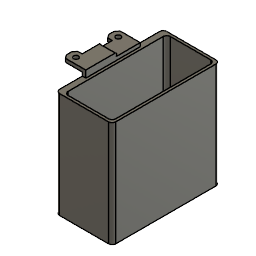
Mounting Bracke_bx_V2 (Autodesk Fusion 360 design; units mm, degrees)
Autodesk Fusion 360 part; units mm, degrees
sketch "Sketch1" plane through (0, 0, 0) normal (0, 1, 0) x (1, 0, 0)
  line L0 (0, 0) -> (0, 24)
  circle A0 centre (0, 24) radius 1.4
  circle A1 centre (0, 0) radius 1.4
  line L1 (0, 0) -> (0, -3.5)
  line L2 (0, 0) -> (0, 3.5)
  line L3 (0, -3.5) -> (-2.5, -3.5)
  line L4 (0, 3.5) -> (-2.5, 3.5)
  line L5 (-4, 0) -> (-4, 1.5)
  line L6 (-4, 0) -> (-4, -1.5)
  line L7 (-2.5, 3.5) -> (-4, 1.5)
  line L8 (-4, -1.5) -> (-2.5, -3.5)
  line L9 (0, 3.5) -> (0, 24)
  line L10 (0, 24) -> (0, 20.5)
  line L11 (0, 24) -> (5, 24)
  line L12 (5, 24) -> (5, 0)
  line L13 (5, 0) -> (0, 0)
  line L14 (5, 12) -> (0, 12)
  line L15 (-2.5, 20.5) -> (-4, 22.5)
  line L16 (0, 20.5) -> (-2.5, 20.5)
  line L17 (-4, 24) -> (-4, 22.5)
  line L18 (-4, 24) -> (-4, 25.5)
  line L19 (0, 27.5) -> (-2.5, 27.5)
  line L20 (-4, 25.5) -> (-2.5, 27.5)
  line L21 (0, -3.5) -> (5, -3.5)
  line L22 (5, -3.5) -> (5, 0)
  line L23 (0, 27.5) -> (5, 27.5)
  line L24 (5, 27.5) -> (5, 24)
  line L25 (0, 27.5) -> (0, 24)
  line L26 (0, 20.5) -> (5, 20.5)
  dimension "d1" = 24
  dimension "d2" = 2.8
  dimension "d3" = 2.8
  dimension "d4" = 3.5
  dimension "d5" = 3.5
  dimension "d6" = 2.5
  dimension "d7" = 2.5
  dimension "d8" = 1.5
  dimension "d9" = 1.5
  dimension "d10" = 3.5
  constraint coincident L0.start A1.centre
  constraint vertical L0
  constraint coincident L0.end A0.centre
  constraint parallel L0 L1
  constraint parallel L0 L2
  constraint perpendicular L1 L3
  constraint perpendicular L2 L4
  constraint vertical L5
  constraint parallel L5 L6
  constraint parallel L9 L10
  constraint perpendicular L10 L11
  constraint perpendicular L11 L12
  constraint perpendicular L1 L13
  constraint midpoint L12 L14.start
  constraint midpoint L0 L14.end
  constraint symmetric L1.end L14 L19.start
  constraint symmetric L2.end L14 L10.end
  constraint symmetric L3.end L14 L19.end
  constraint symmetric L4.end L14 L15.start
  constraint symmetric L5.start L14 L17.start
  constraint symmetric L5.end L14 L15.end
  constraint symmetric L6.end L14 L18.end
  constraint perpendicular L1 L21
  constraint perpendicular L13 L22
  constraint perpendicular L12 L23
  constraint perpendicular L11 L24
  constraint coincident L12 L26.end
  constraint perpendicular L12 L26
  measures "d1" distance of L0.start L0.end
  measures "d2" diameter of A0
  measures "d3" diameter of A1
  measures "d4" distance of L0.start L1.end
  measures "d5" distance of L0.start L2.end
  measures "d6" distance of L1.end L3.end
  measures "d7" distance of L2.end L4.end
  measures "d8" distance of L5.start L5.end
  measures "d9" distance of L5.start L6.end
  measures "d10" distance of L0.end L10.end
extrude "Extrude1" add sketch "Sketch1" along normal blind 2 contours L0 A1 L2 L9 L12 L13 L14 | L0 A1 L1 L2 L3 L4 L5 L6 L7 L8 | L0 L9 L12 L14 L26 | L0 A0 L9 L10 L15 L16 L17 L18 L19 L20 L25 | L0 A0 L9 L10 L11 L12 L26 | A1 L1 L13 L21 L22 | A0 L11 L23 L24 L25
sketch "Sketch2" plane through (0, 2, 0) normal (0, 1, 0) x (-1, 0, 0)
  circle A0 centre (0, 0) radius 1.4
  circle A1 centre (0, -24) radius 1.4
  line L0 (-5, -27.5) -> (2.5, -27.5)
  line L1 (2.5, -27.5) -> (4, -25.5)
  line L2 (4, -25.5) -> (4, -22.5)
  line L3 (4, -22.5) -> (2.5, -20.5)
  line L4 (2.5, -20.5) -> (0, -20.5)
  line L5 (0, -20.5) -> (0, -3.5)
  line L6 (0, -3.5) -> (2.5, -3.5)
  line L7 (2.5, -3.5) -> (4, -1.5)
  line L8 (4, -1.5) -> (4, 1.5)
  line L9 (4, 1.5) -> (2.5, 3.5)
  line L10 (2.5, 3.5) -> (-5, 3.5)
  line L11 (-5, 3.5) -> (-5, -27.5)
  line L12 (0, -15) -> (-5, -15)
  constraint coincident L5 L12.start
  constraint coincident L11 L12.end
  constraint perpendicular L11 L12
extrude "Extrude2" add sketch "Sketch2" along normal blind 2 contours L5 L6 L7 L8 L9 L10 L11 L12
extrude "Extrude3" add 1 faces at (1.6667, 2.6667, -15) along direction (0, 0, -1) blind 5
extrude "Extrude4" add 1 faces at (5, 2, -4.3333) along direction (1, 0, 0) blind 2
fillet "Fillet1" radius 0.75 1 edges at (3.5, 4, -20)
extrude "Extrude5" add 1 faces at (7, 2.6667, -4.0833) along direction (1, 0, 0) blind 2
sketch "Sketch3" plane through (0, 0, 0) normal (0, -1, 0) x (1, 0, 0)
  circle A0 centre (0, 0) radius 1.4
  circle A1 centre (0, -24) radius 1.4
  line L0 (-2.5, -27.5) -> (9, -27.5)
  line L1 (9, -27.5) -> (9, 3.5)
  line L2 (9, 3.5) -> (-2.5, 3.5)
  line L3 (-2.5, 3.5) -> (-4, 1.5)
  line L4 (-4, 1.5) -> (-4, -1.5)
  line L5 (-4, -1.5) -> (-2.5, -3.5)
  line L6 (-2.5, -3.5) -> (0, -3.5)
  line L7 (0, -3.5) -> (0, -20.5)
  line L8 (0, -20.5) -> (-2.5, -20.5)
  line L9 (-2.5, -20.5) -> (-4, -22.5)
  line L10 (-4, -22.5) -> (-4, -25.5)
  line L11 (-4, -25.5) -> (-2.5, -27.5)
  line L12 (9, 3.5) -> (7, 3.5)
  line L13 (7, 3.5) -> (7, -27.5)
  line L14 (7, -27.5) -> (9, -27.5)
  line L15 (9, -27.5) -> (9, 3.5)
  constraint horizontal L12
  constraint vertical L13
  constraint horizontal L14
  constraint vertical L15
  constraint coincident L0 L13.end
  constraint coincident L1.end L2.start
extrude "Extrude6" add sketch "Sketch3" along normal blind 15 contours L0 L1 L2 L12 L13 L14 L15
sketch "Sketch4" plane through (9, 0, 0) normal (1, 0, 0) x (0, 0, -1)
  arc A0 (20, 3.25) -> (19.25, 4) centre (19.25, 3.25) ccw
  line L0 (19.25, 4) -> (-3.5, 4)
  line L1 (-3.5, 4) -> (-3.5, -15)
  line L2 (-3.5, -15) -> (27.5, -15)
  line L3 (27.5, -15) -> (27.5, 2)
  line L4 (27.5, 2) -> (20, 2)
  line L5 (20, 2) -> (20, 3.25)
  line L6 (-3.5, 0) -> (27.5, 0)
  line L7 (27.5, 0) -> (27.5, -15)
  line L8 (27.5, -15) -> (-3.5, -15)
  line L9 (-3.5, -15) -> (-3.5, 0)
  constraint horizontal L6
  constraint vertical L7
  constraint horizontal L8
  constraint vertical L9
  constraint coincident L2.end L3.start
  constraint coincident L1 L6.start
extrude "Extrude7" add sketch "Sketch4" along normal blind 20 contours L1 L2 L3 L6 L7 L8 L9
sketch "Sketch5" plane through (0, 0, 0) normal (0, 1, 0) x (-1, 0, 0)
  line L0 (-9, -27.5) -> (-9, 3.5)
  line L1 (-9, 3.5) -> (-29, 3.5)
  line L2 (-29, 3.5) -> (-29, -27.5)
  line L3 (-29, -27.5) -> (-9, -27.5)
  line L4 (-29, 3.5) -> (-27.5, 3.5)
  line L5 (-27.5, 3.5) -> (-27.5, 2)
  line L6 (-9, -27.5) -> (-10.5, -27.5)
  line L7 (-10.5, -27.5) -> (-10.5, -26)
  line L8 (-27.5, 2) -> (-10.5, 2)
  line L9 (-10.5, 2) -> (-10.5, -26)
  line L10 (-10.5, -26) -> (-27.5, -26)
  line L11 (-27.5, -26) -> (-27.5, 2)
  dimension "d27" = 1.5
  dimension "d28" = 1.5
  dimension "d29" = 1.5
  dimension "d30" = 1.5
  constraint coincident L1.end L2.start
  constraint perpendicular L2 L4
  constraint perpendicular L4 L5
  constraint coincident L0.start L3.end
  constraint perpendicular L0 L6
  constraint perpendicular L6 L7
  constraint horizontal L8
  constraint vertical L9
  constraint horizontal L10
  constraint vertical L11
  measures "d27" distance of L1.end L4.end
  measures "d28" distance of L4.end L5.end
  measures "d29" distance of L0.start L6.end
  measures "d30" distance of L6.end L7.end
extrude "Extrude8" cut sketch "Sketch5" against normal blind 14 contours L8 L9 L10 L11
sketch "Sketch6" plane through (0, 0, 0) normal (0, -1, 0) x (1, 0, 0)
  line L0 (7, -27.5) -> (7, 3.5)
  line L1 (7, 3.5) -> (-2.5, 3.5)
  line L2 (-2.5, 3.5) -> (-4, 1.5)
  line L3 (-4, 1.5) -> (-4, -1.5)
  line L4 (-4, -1.5) -> (-2.5, -3.5)
  line L5 (-2.5, -3.5) -> (0, -3.5)
  line L6 (0, -3.5) -> (0, -20.5)
  line L7 (0, -20.5) -> (-2.5, -20.5)
  line L8 (-2.5, -20.5) -> (-4, -22.5)
  line L9 (-4, -22.5) -> (-4, -25.5)
  line L10 (-4, -25.5) -> (-2.5, -27.5)
  line L11 (-2.5, -27.5) -> (7, -27.5)
  circle A0 centre (0, 0) radius 1.4
  circle A1 centre (0, -24) radius 1.4
  line L12 (0, -11) -> (7, -11)
  constraint coincident L6 L12.start
  constraint coincident L0 L12.end
  constraint perpendicular L0 L12
extrude "Extrude9" cut sketch "Sketch6" against normal blind 2 contours L0 L1 L2 L3 L4 L5 L6 L12
fillet "Fillet2" radius 2 2 edges at (3.5, 0, -11) (3.5, 2, -11)
sketch "Sketch7" plane through (0, 0, 3.5) normal (0, 0, 1) x (1, 0, 0)
  line L0 (-2.5, 2) -> (7, 2)
  line L1 (7, 2) -> (7, -15)
  line L2 (7, -15) -> (29, -15)
  line L3 (29, -15) -> (29, 0)
  line L4 (29, 0) -> (9, 0)
  line L5 (9, 0) -> (9, 4)
  line L6 (9, 4) -> (-2.5, 4)
  line L7 (-2.5, 4) -> (-2.5, 2)
  line L8 (7, 0) -> (29, 0)
  line L9 (29, 0) -> (29, -15)
  line L10 (29, -15) -> (7, -15)
  line L11 (7, -15) -> (7, 0)
  line L12 (9, 0) -> (9, -15)
  constraint horizontal L8
  constraint vertical L9
  constraint horizontal L10
  constraint vertical L11
  constraint coincident L2.end L3.start
  constraint coincident L1 L8.start
  constraint coincident L4.end L5.start
  constraint coincident L10 L12.end
  constraint perpendicular L10 L12
extrude "Extrude10" add sketch "Sketch7" along normal blind 15 contours L1 L2 L8 L10 L11 L12 | L2 L3 L4 L8 L9 L10 L12
sketch "Sketch8" plane through (0, 0, -27.5) normal (0, 0, -1) x (-1, 0, 0)
  line L0 (-7, 0) -> (2.5, 0)
  line L1 (2.5, 0) -> (2.5, 2)
  line L2 (2.5, 2) -> (-9, 2)
  line L3 (-9, 2) -> (-9, 0)
  line L4 (-9, 0) -> (-29, 0)
  line L5 (-29, 0) -> (-29, -15)
  line L6 (-29, -15) -> (-7, -15)
  line L7 (-7, -15) -> (-7, 0)
  line L8 (-7, 0) -> (-29, 0)
  line L9 (-29, 0) -> (-29, -15)
  line L10 (-29, -15) -> (-7, -15)
  line L11 (-7, -15) -> (-7, 0)
  constraint horizontal L8
  constraint vertical L9
  constraint horizontal L10
  constraint vertical L11
  constraint coincident L5.end L6.start
  constraint coincident L0.start L7.end
extrude "Extrude11" add sketch "Sketch8" along normal blind 15 contours L4 L5 L6 L7 L8 L9 L10 L11
extrude "Extrude12" add 1 faces at (29, -5, -22.1667) along direction (1, 0, 0) blind 30
extrude "Extrude13" add 1 faces at (24.3333, -15, -22.1667) along direction (0, -1, 0) blind 45
extrude "Extrude14" cut 1 faces at (21.8333, -4.6667, 2) along direction (0, 0, 1) blind 15
extrude "Extrude15" cut 1 faces at (16.1667, -4.6667, -26) along direction (0, 0, -1) blind 15
extrude "Extrude16" cut 1 faces at (59, -40, -1.8333) along direction (-1, 0, 0) blind 20
extrude "Extrude17" cut 1 faces at (27.5, -9.3333, -2.3333) along direction (1, 0, 0) blind 10
extrude "Extrude18" cut 1 faces at (28.5, -14, -2.3333) along direction (0, -1, 0) blind 44
fillet "Fillet3" radius 2 8 edges at (39, -30, -42.5) (37.5, -29, -41) (37.5, -29, 17) (39, -30, 18.5) (7, -30, 18.5) (10.5, -29, 17) (7, -30, -42.5) (10.5, -29, -41)
sketch "Sketch9" plane through (0, 4, 0) normal (0, 1, 0) x (-1, 0, 0)
  line L0 (-9, -19.25) -> (0, -19.25)
  line L1 (0, -19.25) -> (0, -3.5)
  line L2 (0, -3.5) -> (2.5, -3.5)
  line L3 (2.5, -3.5) -> (4, -1.5)
  line L4 (4, -1.5) -> (4, 1.5)
  line L5 (4, 1.5) -> (2.5, 3.5)
  line L6 (2.5, 3.5) -> (-9, 3.5)
  line L7 (-9, 3.5) -> (-9, -19.25)
  circle A0 centre (0, 0) radius 1.4
  line L8 (0, -15) -> (-9, -15)
  line L9 (-9, -15) -> (-9, -20)
  line L10 (-9, -20) -> (0, -20)
  line L11 (0, -20) -> (0, -15)
  constraint horizontal L8
  constraint vertical L9
  constraint horizontal L10
  constraint vertical L11
  constraint coincident L1 L8.start
extrude "Extrude19" cut sketch "Sketch9" against normal blind 2 contours L0 L1 L7 L8 L9 L11 | L0 L9 L10 L11
extrude "Extrude20" cut 1 faces at (3, 3.3333, -15) along direction (0, 0, 1) blind 1
fillet "Fillet4" radius 0.75 1 edges at (4.5, 4, -14)
